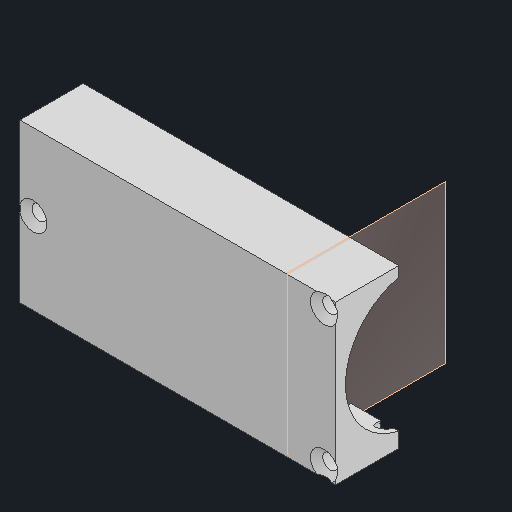
# Autodesk Inventor part: right_motor_ceil
Saved by Autodesk Inventor 2023 (Build 270158000, 158)
## iProperties
Created: 2024-04-24
Part Number: right_motor_ceil
Material: Generic
Document SubType Name: Modeling
Designer: szymo
Density: 1 g/cm^3
Appearance: Default
Author: szymo
Autodesk Inventor part; units mm, degrees
ref_plane "Work Plane1" through (0, -15.375, -1.5) normal (1, 0, 0) x (0, -1, 0)
sketch "Sketch1" plane through (0, -15.375, -1.5) normal (1, 0, 0) x (0, -1, 0)
  circle A0 centre (8, 0) radius 1.0564 projected
  circle A1 centre (-8, 0) radius 1.0564 projected
  circle A2 centre (0, 0) radius 5 projected
  circle A3 centre (0, 0) radius 13.7 projected
  line L0 (16.375, -1.5) -> (9.8735, -1.5) projected
  line L1 (16.375, -1.5) -> (16.375, 15.375) projected
  line L2 (16.375, 15.375) -> (-15.375, 15.375) projected
  line L3 (-15.375, 15.375) -> (-15.375, -1.5) projected
  line L4 (-15.375, -1.5) -> (-9.8735, -1.5) projected
  arc A4 (-6.7025, 2.019) -> (-9.8735, -1.5) centre (-8, 0) ccw projected
  arc A5 (6.7025, 2.019) -> (-6.7025, 2.019) centre (0, 0) ccw projected
  arc A6 (9.8735, -1.5) -> (6.7025, 2.019) centre (8, 0) ccw projected
  line L5 (16.375, -15.7) -> (-15.375, -15.7)
  line L6 (-15.375, -15.7) -> (-15.375, -3)
  line L7 (-15.375, -3) -> (16.375, -3)
  line L8 (16.375, -3) -> (16.375, -15.7)
  point P0 (0, -13.7)
  point P1 (13.3675, -3)
  point P2 (-13.3675, -3)
  dimension "d0" = 1.5
  dimension "d1" = 2
  constraints: 8 end point, 2 collinear, 2 parallel, 1 horizontal, 1 perpendicular, 3 other
  measures "d0" distance between parallel lines of L7 L0
  measures "d1" distance from line of L5 point (0, -13.7)
ref_plane "Work Plane2" through (9.5, -31.75, -16.875) normal (1, 0, 0) x (0, 1, 0)
extrude "Extrusion1" add sketch "Sketch1" along normal up to surface (9.5 mm away) contours A3 L7 L8 L5 L6
sketch "Sketch2" plane through (0, -15.375, -1.5) normal (-1, 0, 0) x (0, 0, 1)
  circle A0 centre (0, 0) radius 14.375 projected
  line L0 (15.7, 15.375) -> (15.7, -16.375) projected
  line L1 (3, 15.375) -> (15.7, 15.375) projected
  line L2 (3, 13.3675) -> (3, 15.375) projected
  arc A1 (3, -13.3675) -> (3, 13.3675) centre (0, 0) ccw projected
  line L3 (3, -16.375) -> (3, -13.3675) projected
  line L4 (15.7, -16.375) -> (3, -16.375) projected
  point P0 (1.5, 15.375)
  point P1 (3, 14.0585)
  point P2 (3, -14.0585)
ref_plane "Work Plane3" through (-27.7, -29.75, -15.875) normal (-1, 0, 0) x (0, 0, 1)
extrude "Extrusion2" add sketch "Sketch2" along normal up to surface (27.7 mm away) contours A0 L2 L1 L0 L4 L3
sketch "Sketch3" plane through (-27.7, -15.375, -1.5) normal (-1, 0, 0) x (0, 0, 1)
  line L0 (-1.5, 11) -> (-1.5, 11.5) projected
  line L1 (-1.5, 11.5) -> (1.5, 11.5) projected
  line L2 (1.5, 11.5) -> (1.5, 11) projected
  line L3 (1.5, 11) -> (-1.5, 11) projected
  line L4 (1.5, -11.5) -> (1.5, -12) projected
  line L5 (1.5, -12) -> (-1.5, -12) projected
  line L6 (-1.5, -12) -> (-1.5, -11.5) projected
  line L7 (-1.5, -11.5) -> (1.5, -11.5) projected
  circle A0 centre (0, 0) radius 5 projected
  circle A1 centre (0, 0) radius 13.7 projected
  line L8 (15.7, -16.375) -> (3, -16.375) projected
  line L9 (15.7, 15.375) -> (15.7, -16.375) projected
  line L10 (3, 15.375) -> (15.7, 15.375) projected
  line L11 (3, 14.0585) -> (3, 15.375) projected
  arc A2 (3, -14.0585) -> (3, 14.0585) centre (0, 0) ccw projected
  line L12 (3, -16.375) -> (3, -14.0585) projected
  circle A3 centre (0, 0) radius 14.375 projected
  circle A4 centre (0, 0) radius 13.7 projected
  line L13 (15.7, 15.375) -> (3, 15.375) projected
  line L14 (15.7, 15.375) -> (3, 15.375)
  line L15 (3, 15.375) -> (3, -16.375)
  line L16 (3, -16.375) -> (15.7, -16.375)
  line L17 (15.7, -16.375) -> (15.7, 15.375)
  point P0 (1.5, 15.375)
  point P1 (3, -13.3675)
  point P2 (3, -14.0585)
  point P3 (3, 13.3675)
  constraints: 8 end point, 2 parallel, 1 horizontal, 1 perpendicular
ref_plane "Work Plane4" through (-41.5, -31.75, -7.5) normal (-1, 0, 0) x (0, 0, 1)
extrude "Extrusion3" add sketch "Sketch3" along normal up to surface (13.8 mm away) contours L15 A2 A1 | L11 L10 L9 L8 L12 A2
sketch "Sketch4" plane through (-41.5, -15.375, -1.5) normal (-1, 0, 0) x (0, 0, 1)
  arc A0 (3, -13.3675) -> (3, 13.3675) centre (0, 0) ccw projected
  line L0 (3, -16.375) -> (3, -13.3675) projected
  line L1 (15.7, -16.375) -> (3, -16.375) projected
  line L2 (15.7, 15.375) -> (15.7, -16.375) projected
  line L3 (3, 15.375) -> (15.7, 15.375) projected
  line L4 (3, 13.3675) -> (3, 15.375) projected
  line L5 (15.7, 15.375) -> (3, 15.375) projected
  line L6 (3, -16.375) -> (15.7, -16.375) projected
  line L7 (15.7, 15.375) -> (9.7, 15.375)
  line L8 (9.7, 15.375) -> (9.7, -16.375)
  line L9 (9.7, -16.375) -> (15.7, -16.375)
  line L10 (15.7, -16.375) -> (15.7, 15.375)
  point P0 (1.5, 15.375)
  point P1 (9.7, -9.6747)
  point P2 (9.7, -16.375)
  dimension "d8" = 6
  constraints: 8 end point, 2 parallel, 1 horizontal, 1 perpendicular, 1 point on line
  measures "d8" distance of L9.end L8.end
ref_plane "Work Plane5" through (-48.5, -20.375, -7.5) normal (1, 0, 0) x (0, 1, 0)
extrude "Extrusion4" add sketch "Sketch4" along normal up to surface (7 mm away) contours A0 L8 L3 L2 L1 | A0 L4 L3 L8
sketch "Sketch5" plane through (-48.5, -31.75, 14.2) normal (-1, 0, 0) x (0, 0, 1)
  line L0 (-12.7, 31.75) -> (-12.7, 29.7425) projected
  arc A0 (-6, 6.7003) -> (-12.7, 29.7425) centre (-15.7, 16.375) ccw projected
  line L1 (-6, 6.7003) -> (-6, 0) projected
  line L2 (-6, 0) -> (0, 0) projected
  line L3 (0, 0) -> (0, 31.75) projected
  line L4 (0, 31.75) -> (-12.7, 31.75) projected
  line L5 (-6, 0) -> (-6, 6.7003) projected
  arc A1 (-12.7, 3.0075) -> (-6, 6.7003) centre (-15.7, 16.375) ccw projected
  line L6 (-12.7, 0) -> (-12.7, 3.0075) projected
  line L7 (-6, 0) -> (-12.7, 0) projected
  line L8 (0, 0) -> (0, 31.75) projected
  line L9 (-12.7, 0) -> (0, 0) projected
  line L10 (0, 31.75) -> (-12.7, 31.75)
  line L11 (-12.7, 31.75) -> (-12.7, 0)
  line L12 (-12.7, 0) -> (0, 0)
  line L13 (0, 0) -> (0, 31.75)
  line L14 (-6, 6.7003) -> (-12.7, 6.7003)
  point P0 (-14.2, 31.75)
  point P1 (-6, 6.7003)
  constraints: 10 end point, 2 parallel, 2 perpendicular, 1 horizontal, 1 point on line
ref_plane "Work Plane6" through (-53.8, -31.75, -16.875) normal (-1, 0, 0) x (0, 0, 1)
extrude "Extrusion5" add sketch "Sketch5" along normal up to surface (5.3 mm away) contours L4 L3 L2 L1 A0 L0 | A0 L14 L11
sketch "Sketch6" plane through (9.5, -31.75, 14.2) normal (0, 0, 1) x (1, 0, 0)
  circle A0 centre (-2.3, 29.45) radius 1.55 projected
  circle A1 centre (-2.3, 2.3) radius 1.55 projected
  circle A2 centre (-60.65, 16.375) radius 1.55 projected
  point P0 (-9.5, 31.75)
  constraints: 3 coincident
hole "Hole1" at (7.2, -2.3, 14.2) at (7.2, -29.45, 14.2) at (-51.15, -15.375, 14.2) direction (0, 0, -1) diameter 3 depth 14.5 countersink diameter 5.5 countersink angle 90 clearance for "Countersunk Flat Head Screw ISO 2009/7046" size "M2.5" standard "ISO"
body "Solid1"
